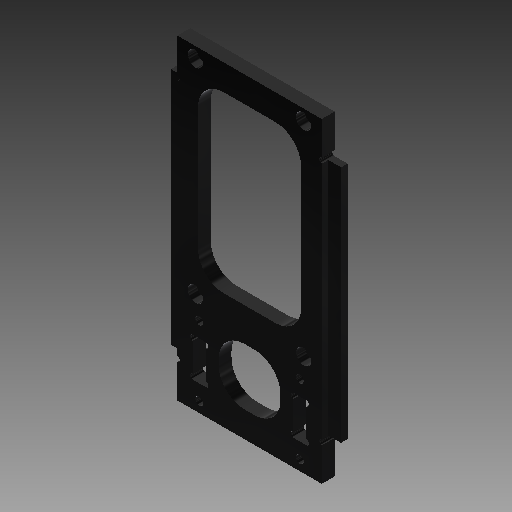
# Autodesk Inventor part: コックピット_2_サブフレーム_2
Saved by Autodesk Inventor 2018 (Build 220112000, 112)
## iProperties
Category: コックピット
Created: 2016-05-24
Part Number: コックピット_2_サブフレーム_2
Material: アセタール樹脂、黒
Document SubType Name: Modeling
Designer: hiroaki
Density: 1.425 g/cm^3
Appearance: 滑らか - 黒
Mass: 28.3031 g
Surface Area: 131.763 cm^2
Volume: 19.8619 cm^3
Author: hiroaki
Autodesk Inventor part; units mm, degrees
ref_plane "YZ Plane" through (0, 0, 0) normal (1, 0, 0) x (0, 1, 0)
ref_plane "XZ Plane" through (0, 0, 0) normal (0, 1, 0) x (-1, 0, 0)
ref_plane "XY Plane" through (0, 0, 0) normal (0, 0, 1) x (1, 0, 0)
sketch "スケッチ1" plane through (0, 0, 0) normal (0, 0, 1) x (1, 0, 0)
  line L0 (-28, -61.25) -> (28, -61.25) construction
  line L1 (28, -61.25) -> (28, 61.25) construction
  line L2 (28, 61.25) -> (-28, 61.25) construction
  line L3 (-28, 61.25) -> (-28, -61.25) construction
  line L4 (-28, -61.25) -> (28, 61.25) construction
  line L5 (28, -61.25) -> (-28, 61.25) construction
  line L6 (-28, 48.35) -> (-28, 61.25)
  line L7 (-28, 61.25) -> (28, 61.25)
  line L8 (28, 61.25) -> (28, 48.35)
  line L9 (-28, 46.25) -> (-33, 46.25)
  line L10 (-33, 46.25) -> (-33, -46.25)
  line L11 (-33, -46.25) -> (-28, -46.25)
  line L12 (-28, -48.35) -> (-28, -61.25)
  line L13 (-28, -61.25) -> (28, -61.25)
  line L14 (28, -61.25) -> (28, -48.35)
  line L15 (28, 46.25) -> (33, 46.25)
  line L16 (33, 46.25) -> (33, -46.25)
  line L17 (33, -46.25) -> (28, -46.25)
  arc A0 (-28, 46.25) -> (-28, 48.35) centre (-28, 47.3) ccw
  arc A1 (-28, -48.35) -> (-28, -46.25) centre (-28, -47.3) ccw
  arc A2 (28, -46.25) -> (28, -48.35) centre (28, -47.3) ccw
  line L18 (0, 0) -> (0, 61.25) construction
  line L19 (0, 0) -> (28, 0) construction
  arc A3 (28, 48.35) -> (28, 46.25) centre (28, 47.3) ccw
  line L20 (-21, 56.95) -> (21, 56.95) construction
  line L21 (21, 56.95) -> (21, -22.05) construction
  line L22 (21, -22.05) -> (-21, -22.05) construction
  line L23 (-21, -22.05) -> (-21, 56.95) construction
  line L24 (-21, 56.95) -> (21, -22.05) construction
  line L25 (21, 56.95) -> (-21, -22.05) construction
  circle A4 centre (-21, 56.95) radius 1.6
  circle A5 centre (-21, -22.05) radius 1.6
  circle A6 centre (21, -22.05) radius 1.6
  circle A7 centre (21, 56.95) radius 1.6
  line L26 (-22, -36.25) -> (-17, -36.25) construction
  line L27 (-17, -36.25) -> (-17, -51.25) construction
  line L28 (-17, -51.25) -> (-22, -51.25) construction
  line L29 (-22, -51.25) -> (-22, -36.25) construction
  circle A8 centre (-19.5, -30.25) radius 1.55
  circle A9 centre (-19.5, -57.25) radius 1.55
  line L30 (-17, -43.75) -> (-22, -43.75) construction
  line L31 (-22, -26.25) -> (-17, -26.25) construction
  line L32 (-17, -26.25) -> (-17, -61.25) construction
  line L33 (-17, -61.25) -> (-22, -61.25) construction
  line L34 (-22, -61.25) -> (-22, -26.25) construction
  circle A10 centre (-19.5, -57.25) radius 3 construction
  line L35 (-16.95, -36.2) -> (-22.05, -36.2)
  line L36 (-22.05, -36.2) -> (-22.05, -51.3)
  line L37 (-22.05, -51.3) -> (-16.95, -51.3)
  line L38 (-16.95, -51.3) -> (-16.95, -36.2)
  circle A11 centre (-22.05, -37.25) radius 1.05
  circle A12 centre (-16.95, -37.25) radius 1.05
  circle A13 centre (-22.05, -50.25) radius 1.05
  circle A14 centre (-16.95, -50.25) radius 1.05
  circle A15 centre (19.5, -30.25) radius 1.55
  circle A16 centre (19.5, -57.25) radius 1.55
  line L39 (16.95, -36.2) -> (22.05, -36.2)
  line L40 (22.05, -36.2) -> (22.05, -51.3)
  line L41 (22.05, -51.3) -> (16.95, -51.3)
  line L42 (16.95, -51.3) -> (16.95, -36.2)
  circle A17 centre (22.05, -37.25) radius 1.05
  circle A18 centre (16.95, -37.25) radius 1.05
  circle A19 centre (22.05, -50.25) radius 1.05
  circle A20 centre (16.95, -50.25) radius 1.05
  point P0 (0, 17.45)
  point P1 (0, 17.45)
  point P2 (0, 0)
  point P3 (-19.5, -43.75)
  point P4 (-19.5, -26.25)
  dimension "d93" = 2.1
  dimension "d9" = 56
  dimension "d12" = 122.5
  dimension "d13" = 15
  dimension "d39" = 15
  dimension "d40" = 1.05
  dimension "d41" = 5
  dimension "d52" = 3.2
  dimension "d53" = 42
  dimension "d54" = 79
  dimension "d55" = 4.3
  dimension "d73" = 35
  dimension "d83" = 5
  dimension "d87" = 3.1
  dimension "d88" = 10
  dimension "d89" = 27
  dimension "d90" = 6
  dimension "d91" = 22
  dimension "d92" = 0.05
  constraints: 86 end point, 16 symmetric about line, 14 perpendicular, 13 centre point, 13 midpoint, 12 point on line, 12 vertical alignment, 10 parallel, 8 point on circle, 6 collinear, 6 horizontal, 6 vertical, 5 coincident, 5 equal radius, 3 horizontal alignment, 1 tangent, 22 other
  measures "d9" distance of L1.end L2.end
  measures "d12" distance of L0.end L1.end
  measures "d13" distance between parallel lines of L9 L2
  measures "d39" distance between parallel lines of L0 L11
  measures "d40" radius of A0
  measures "d41" distance of L9.start L9.end
  measures "d52" diameter of A4
  measures "d53" distance of L20.start L20.end
  measures "d54" distance of L22.end L20.start
  measures "d55" distance between parallel lines of L2 L20
  measures "d73" distance of L31.end L32.end
  measures "d83" distance of L31.start L31.end
  measures "d87" diameter of A8
  measures "d88" distance between parallel lines of L31 L26
  measures "d89" distance of A9.centre A8.centre
  measures "d90" diameter of A10
  measures "d91" distance between parallel lines of L18 L34
  measures "d92" distance between parallel lines of L35 L26
extrude "押し出し1" add sketch "スケッチ1" along normal blind 5
sketch "スケッチ2" plane through (0, 0, 5) normal (0, 0, 1) x (1, 0, 0)
  line L0 (-28, 61.25) -> (-28, 48.35) projected
  line L1 (28, 61.25) -> (-28, 61.25) projected
  line L2 (-67.7785, 47.5) -> (-28, 47.5)
  line L3 (-28, 47.5) -> (-28, -47.5)
  line L4 (-28, -47.5) -> (-67.7785, -47.5)
  line L5 (-67.7785, -47.5) -> (-67.7785, 47.5)
  line L6 (67.7785, 47.5) -> (28, 47.5)
  line L7 (28, 47.5) -> (28, -47.5)
  line L8 (28, -47.5) -> (67.7785, -47.5)
  line L9 (67.7785, -47.5) -> (67.7785, 47.5)
  line L10 (0, 0) -> (0, 61.25) construction
  line L11 (0, 0) -> (33, 0) construction
  line L12 (33, 46.25) -> (33, -46.25) construction
  dimension "d106" = 95
  constraints: 20 end point, 4 parallel, 2 horizontal, 2 midpoint, 2 perpendicular, 2 symmetric about line, 1 collinear, 3 other
  measures "d106" distance between parallel lines of L4 L2
extrude "押し出し2" cut sketch "スケッチ2" against normal blind 2.5
sketch "スケッチ4" plane through (0, 0, 5) normal (0, 0, 1) x (1, 0, 0)
  line L0 (28, 61.25) -> (-28, 61.25) projected
  line L1 (-28, 61.25) -> (-28, 48.35) projected
  line L2 (-28, -61.25) -> (28, -61.25) projected
  line L3 (-16.95, -51.3) -> (-22.05, -51.3) projected
  arc A0 (-22.05, -49.2) -> (-22.05, -51.3) centre (-22.05, -50.25) ccw projected
  line L4 (-22.05, -49.2) -> (-22.05, -38.3) projected
  arc A1 (-22.05, -36.2) -> (-22.05, -38.3) centre (-22.05, -37.25) ccw projected
  line L5 (-22.05, -36.2) -> (-16.95, -36.2) projected
  arc A2 (-16.95, -38.3) -> (-16.95, -36.2) centre (-16.95, -37.25) ccw projected
  line L6 (-16.95, -38.3) -> (-16.95, -49.2) projected
  arc A3 (-16.95, -51.3) -> (-16.95, -49.2) centre (-16.95, -50.25) ccw projected
  circle A4 centre (-19.5, -30.25) radius 1.55 projected
  line L7 (-20, 51.25) -> (20, 51.25)
  line L8 (20, 51.25) -> (20, -16.25)
  line L9 (20, -16.25) -> (-20, -16.25)
  line L10 (-20, -16.25) -> (-20, 51.25)
  line L11 (-12, -29.25) -> (12, -29.25)
  line L12 (12, -29.25) -> (12, -51.25)
  line L13 (12, -51.25) -> (-12, -51.25)
  line L14 (-12, -51.25) -> (-12, -29.25)
  line L15 (-16.95, -36.25) -> (-22.05, -36.25) construction
  arc A5 (-22.05, -36.25) -> (-22, -38.2487) centre (-22.05, -37.25) ccw construction
  line L16 (-22, -38.2487) -> (-22, -49.2513) construction
  arc A6 (-22, -49.2513) -> (-22.05, -51.25) centre (-22.05, -50.25) ccw construction
  line L17 (-22.05, -51.25) -> (-16.95, -51.25) construction
  arc A7 (-16.95, -51.25) -> (-17, -49.2513) centre (-16.95, -50.25) ccw construction
  line L18 (-17, -49.2513) -> (-17, -38.2487) construction
  arc A8 (-17, -38.2487) -> (-16.95, -36.25) centre (-16.95, -37.25) ccw construction
  point P0 (0, 0)
  point P1 (0, 51.25)
  point P2 (0, -16.25)
  point P3 (0, -29.25)
  dimension "d94" = 8
  dimension "d95" = 10
  dimension "d96" = 14
  dimension "d97" = 0.05
  dimension "d98" = 5
  dimension "d99" = 10
  dimension "d100" = 13
  constraints: 24 end point, 8 point on circle, 4 centre point, 4 parallel, 3 midpoint, 2 horizontal, 2 perpendicular, 2 vertical alignment, 7 other
  measures "d94" distance between parallel lines of L1 L10
  measures "d95" distance between parallel lines of L0 L7
  measures "d96" distance from line of A4.centre L9
  measures "d97" distance between parallel lines of L6 L18
  measures "d98" distance between parallel lines of L14 L18
  measures "d99" distance between parallel lines of L2 L13
  measures "d100" distance between parallel lines of L9 L11
extrude "押し出し4" cut sketch "スケッチ4" against normal blind 10 contours L7 L8 L9 L10 | L11 L12 L13 L14
fillet "フィレット2" radius 10 8 edges at (-12, -51.25, 2.5) (-12, -29.25, 2.5) (12, -29.25, 2.5) (12, -51.25, 2.5) (-20, -16.25, 2.5) (-20, 51.25, 2.5) (20, 51.25, 2.5) (20, -16.25, 2.5)
sketch "スケッチ6" plane through (0, 0, 5) normal (0, 0, 1) x (1, 0, 0)
  circle A0 centre (-21, 57) radius 3
  circle A1 centre (-21, -22) radius 3
  line L0 (0, 0) -> (0, 20)
  circle A2 centre (21, 57) radius 3
  circle A3 centre (21, -22) radius 3
  dimension "d107" = 6
  dimension "d108" = 6
  dimension "d109" = 79
  dimension "d110" = 57
  dimension "d111" = 21
  dimension "d112" = 20
  constraints: 4 centre point, 2 end point, 2 symmetric about line, 1 vertical, 2 other
  measures "d107" diameter of A0
  measures "d108" diameter of A1
  measures "d109" distance of A0.centre A1.centre
  measures "d110" vertical distance of A0.centre L0.start
  measures "d111" horizontal distance of L0.start A0.centre
  measures "d112" distance of L0.start L0.end
extrude "押し出し5" cut sketch "スケッチ6" against normal blind 3.5
equation "\"d12\" = d19"
equation "\"d13\" = d26"
equation "\"d39\" = d27"
equation "\"d73\" = d1_1_2_3 + 2 * d2_1"
equation "\"d88\" = d2_1"
equation "\"d99\" = d95"
equation "\"d19\" = 122.5"
equation "\"d26\" = 15"
equation "\"d27\" = 15"
equation "\"d1_1_2_3\" = 15"
equation "\"d2_1\" = 10"
